Autodesk Inventor part; units mm, degrees
(part 2 of 2)
  circle A471 centre (-42.6888, 38.1375) radius 0.851
  circle A472 centre (-38.2437, 19.0875) radius 1.994
  circle A473 centre (-43.3237, 19.0875) radius 0.851
  circle A474 centre (-33.1638, 19.0875) radius 0.851
  circle A475 centre (-33.4813, 0.0375) radius 1.994
  circle A476 centre (-38.5613, 0.0375) radius 0.851
  circle A477 centre (-28.4013, 0.0375) radius 0.851
  circle A478 centre (-23.9563, -19.0125) radius 1.994
  circle A479 centre (-29.0362, -19.0125) radius 0.851
  circle A480 centre (-18.8762, -19.0125) radius 0.851
  circle A481 centre (-135.875, 0.0375) radius 1.994
  circle A482 centre (-140.955, 0.0375) radius 0.851
  circle A483 centre (-130.795, 0.0375) radius 0.851
  circle A484 centre (-28.7188, 38.1375) radius 1.994
  circle A485 centre (-33.7987, 38.1375) radius 0.851
  circle A486 centre (-23.6388, 38.1375) radius 0.851
  circle A487 centre (-19.1938, 19.0875) radius 1.994
  circle A488 centre (-24.2737, 19.0875) radius 0.851
  circle A489 centre (-14.1137, 19.0875) radius 0.851
  circle A490 centre (-14.4313, 0.0375) radius 1.994
  circle A491 centre (-19.5113, 0.0375) radius 0.851
  circle A492 centre (-9.3513, 0.0375) radius 0.851
  circle A493 centre (-4.9062, -19.0125) radius 1.994
  circle A494 centre (-9.9863, -19.0125) radius 0.851
  circle A495 centre (0.1737, -19.0125) radius 0.851
  circle A496 centre (-21.575, -38.0625) radius 1.994
  circle A497 centre (-26.655, -38.0625) radius 0.851
  circle A498 centre (-16.495, -38.0625) radius 0.851
  circle A499 centre (-71.613, -31.0775) radius 1.524
  circle A500 centre (28.463, -31.0775) radius 1.524
  circle A501 centre (-71.613, -46.3175) radius 1.994
  circle A502 centre (28.463, -46.3175) radius 1.994
  circle A503 centre (-9.6687, 38.1375) radius 1.994
  circle A504 centre (-14.7487, 38.1375) radius 0.851
  circle A505 centre (-4.5888, 38.1375) radius 0.851
  circle A506 centre (-0.1437, 19.0875) radius 1.994
  circle A507 centre (-5.2238, 19.0875) radius 0.851
  circle A508 centre (4.9363, 19.0875) radius 0.851
  circle A509 centre (4.6188, 0.0375) radius 1.994
  circle A510 centre (-0.4612, 0.0375) radius 0.851
  circle A511 centre (9.6988, 0.0375) radius 0.851
  circle A512 centre (14.1438, -19.0125) radius 1.994
  circle A513 centre (9.0638, -19.0125) radius 0.851
  circle A514 centre (19.2237, -19.0125) radius 0.851
  circle A515 centre (-131.1125, -19.0125) radius 1.994
  circle A516 centre (-136.1925, -19.0125) radius 0.851
  circle A517 centre (-126.0325, -19.0125) radius 0.851
  circle A518 centre (-143.0505, -12.0275) radius 1.524
  circle A519 centre (-119.1745, -12.0275) radius 1.524
  circle A520 centre (-143.0505, -27.2675) radius 1.994
  circle A521 centre (-119.1745, -27.2675) radius 1.994
  circle A522 centre (9.3812, 38.1375) radius 1.994
  circle A523 centre (4.3012, 38.1375) radius 0.851
  circle A524 centre (14.4613, 38.1375) radius 0.851
  circle A525 centre (18.9062, 19.0875) radius 1.994
  circle A526 centre (13.8262, 19.0875) radius 0.851
  circle A527 centre (23.9862, 19.0875) radius 0.851
  circle A528 centre (23.6687, 0.0375) radius 1.994
  circle A529 centre (18.5888, 0.0375) radius 0.851
  circle A530 centre (28.7488, 0.0375) radius 0.851
  circle A531 centre (33.1938, -19.0125) radius 1.994
  circle A532 centre (28.1137, -19.0125) radius 0.851
  circle A533 centre (38.2737, -19.0125) radius 0.851
  circle A534 centre (28.4313, 38.1375) radius 1.994
  circle A535 centre (23.3513, 38.1375) radius 0.851
  circle A536 centre (33.5112, 38.1375) radius 0.851
  circle A537 centre (37.9562, 19.0875) radius 1.994
  circle A538 centre (32.8762, 19.0875) radius 0.851
  circle A539 centre (43.0363, 19.0875) radius 0.851
  circle A540 centre (42.7188, 0.0375) radius 1.994
  circle A541 centre (37.6388, 0.0375) radius 0.851
  circle A542 centre (47.7987, 0.0375) radius 0.851
  circle A543 centre (52.2438, -19.0125) radius 1.994
  circle A544 centre (47.1638, -19.0125) radius 0.851
  circle A545 centre (57.3238, -19.0125) radius 0.851
  circle A546 centre (-140.6375, -38.0625) radius 1.994
  circle A547 centre (-145.7175, -38.0625) radius 0.851
  circle A548 centre (-135.5575, -38.0625) radius 0.851
  circle A549 centre (47.4813, 38.1375) radius 1.994
  circle A550 centre (42.4012, 38.1375) radius 0.851
  circle A551 centre (52.5613, 38.1375) radius 0.851
  circle A552 centre (57.0063, 19.0875) radius 1.994
  circle A553 centre (51.9263, 19.0875) radius 0.851
  circle A554 centre (62.0863, 19.0875) radius 0.851
  circle A555 centre (61.7687, 0.0375) radius 1.994
  circle A556 centre (56.6887, 0.0375) radius 0.851
  circle A557 centre (66.8487, 0.0375) radius 0.851
  circle A558 centre (71.2938, -19.0125) radius 1.994
  circle A559 centre (66.2138, -19.0125) radius 0.851
  circle A560 centre (76.3738, -19.0125) radius 0.851
  circle A561 centre (47.4813, -38.0625) radius 1.994
  circle A562 centre (42.4012, -38.0625) radius 0.851
  circle A563 centre (52.5613, -38.0625) radius 0.851
  circle A564 centre (66.5312, 38.1375) radius 1.994
  circle A565 centre (61.4513, 38.1375) radius 0.851
  circle A566 centre (71.6112, 38.1375) radius 0.851
  circle A567 centre (76.0563, 19.0875) radius 1.994
  circle A568 centre (70.9762, 19.0875) radius 0.851
  circle A569 centre (81.1363, 19.0875) radius 0.851
  circle A570 centre (80.8187, 0.0375) radius 1.994
  circle A571 centre (75.7387, 0.0375) radius 0.851
  circle A572 centre (85.8988, 0.0375) radius 0.851
  circle A573 centre (97.4875, -19.0125) radius 1.994
  circle A574 centre (92.4075, -19.0125) radius 0.851
  circle A575 centre (102.5675, -19.0125) radius 0.851
  circle A576 centre (-123.9688, 38.1375) radius 1.994
  circle A577 centre (-129.0488, 38.1375) radius 0.851
  circle A578 centre (-118.8888, 38.1375) radius 0.851
  circle A579 centre (66.5312, -38.0625) radius 1.994
  circle A580 centre (61.4513, -38.0625) radius 0.851
  circle A581 centre (71.6112, -38.0625) radius 0.851
  circle A582 centre (85.5813, 38.1375) radius 1.994
  circle A583 centre (80.5012, 38.1375) radius 0.851
  circle A584 centre (90.6612, 38.1375) radius 0.851
  circle A585 centre (95.1063, 19.0875) radius 1.994
  circle A586 centre (90.0263, 19.0875) radius 0.851
  circle A587 centre (100.1863, 19.0875) radius 0.851
  circle A588 centre (111.775, 0.0375) radius 1.994
  circle A589 centre (106.695, 0.0375) radius 0.851
  circle A590 centre (116.855, 0.0375) radius 0.851
  circle A591 centre (99.837, 7.0225) radius 1.524
  circle A592 centre (123.713, 7.0225) radius 1.524
  circle A593 centre (99.837, -8.2175) radius 1.994
  circle A594 centre (123.713, -8.2175) radius 1.994
  circle A595 centre (123.6813, -19.0125) radius 1.994
  circle A596 centre (118.6012, -19.0125) radius 0.851
  circle A597 centre (128.7612, -19.0125) radius 0.851
  circle A598 centre (85.5813, -38.0625) radius 1.994
  circle A599 centre (80.5012, -38.0625) radius 0.851
  circle A600 centre (90.6612, -38.0625) radius 0.851
  circle A601 centre (114.1562, 38.1375) radius 1.994
  circle A602 centre (109.0763, 38.1375) radius 0.851
  circle A603 centre (119.2363, 38.1375) radius 0.851
  circle A604 centre (102.2183, 45.1225) radius 1.524
  circle A605 centre (126.0943, 45.1225) radius 1.524
  circle A606 centre (102.2183, 29.8825) radius 1.994
  circle A607 centre (126.0943, 29.8825) radius 1.994
  circle A608 centre (118.9188, 19.0875) radius 1.994
  circle A609 centre (113.8388, 19.0875) radius 0.851
  circle A610 centre (123.9988, 19.0875) radius 0.851
  circle A611 centre (142.7312, 0.0375) radius 1.994
  circle A612 centre (137.6513, 0.0375) radius 0.851
  circle A613 centre (147.8113, 0.0375) radius 0.851
  circle A614 centre (142.7312, -19.0125) radius 1.994
  circle A615 centre (137.6513, -19.0125) radius 0.851
  circle A616 centre (147.8113, -19.0125) radius 0.851
  circle A617 centre (-114.4438, 19.0875) radius 1.994
  circle A618 centre (-119.5238, 19.0875) radius 0.851
  circle A619 centre (-109.3637, 19.0875) radius 0.851
  circle A620 centre (123.6813, -38.0625) radius 1.994
  circle A621 centre (118.6012, -38.0625) radius 0.851
  circle A622 centre (128.7612, -38.0625) radius 0.851
  circle A623 centre (142.7312, 38.1375) radius 1.994
  circle A624 centre (137.6513, 38.1375) radius 0.851
  circle A625 centre (147.8113, 38.1375) radius 0.851
  circle A626 centre (142.7312, 19.0875) radius 1.994
  circle A627 centre (137.6513, 19.0875) radius 0.851
  circle A628 centre (147.8113, 19.0875) radius 0.851
  circle A629 centre (104.6312, -38.0625) radius 1.994
  circle A630 centre (99.5513, -38.0625) radius 0.851
  circle A631 centre (109.7113, -38.0625) radius 0.851
  circle A632 centre (142.7312, -38.0625) radius 1.994
  circle A633 centre (137.6513, -38.0625) radius 0.851
  circle A634 centre (147.8113, -38.0625) radius 0.851
  circle A635 centre (-109.6813, 0.0375) radius 1.994
  circle A636 centre (-114.7613, 0.0375) radius 0.851
  circle A637 centre (-104.6012, 0.0375) radius 0.851
  circle A638 centre (-100.1562, -19.0125) radius 1.994
  circle A639 centre (-105.2363, -19.0125) radius 0.851
  circle A640 centre (-95.0763, -19.0125) radius 0.851
  constraints: 641 centre point, 584 end point, 560 point on circle
extrude "60pc_pcb.kicad_v1.1_pcb.kicad_pcb_Outline" add sketch "Sketch1" along normal blind 1.6
body "Solid1"
